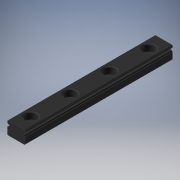
# Autodesk Inventor part: C-MLG9-75_r
Saved by Autodesk Inventor 2019 (Build 230136000, 136)
## iProperties
Created: 2023-11-06
Part Number: C-MLG9-75_r
Material: Generic
Catalog Web Link: www.cadenas.de
Description: C-MLG, E-GMLG_rail-Economy Miniature Liner guide - Standard type
Vendor: MISUMI
Document SubType Name: Modeling
Designer: psAdmin
Manufacturer: MISUMI
Mass: 3.65448 g
Surface Area: 29.3453 cm^2
Volume: 3.65448 cm^3
Density: 1 g/cm^3
Appearance: PSOLRGB-175-175-175
Category: PARTsolutions
Company: MISUMI
Title: C-MLG9-75
Author: Cadenas PARTsolutions
Comments: Economy Miniature Liner guide - Standard type
PSOL_IDENT_0: {$CADENAS_DATA/23d-libs/misumi/metric/06_linear_guides/c_mlg/c_mlg_rail.prj},214 {VTYP=3D},{NB=C-MLG
PSOL_IDENT_1: 9-75_r},{LINA=C-MLG9-75},{NN=C-MLG, E-GMLG_rail},{DATE=31.10.2023 10:57:24},{GEOMDATE=24.08.2023 00:
PSOL_IDENT_2: 31:00},{VERSION=},{LINEID=20},{WBVAR=ST,L,ALT1,ALT2,ALT3,ALT4,ES,ALT5,EB},{WBNUMERIC=L,ES,EB}  {NB=C
PSOL_IDENT_3: -MLG9-75_r},{LINA=C-MLG9-75},{KT=DUMMY},{PN=C-MLG9-75},{TYPE=C-MLG},{ST=1},{NM=9},{L=75},{LALG=[35:9
PSOL_IDENT_4: 00/1]},{H=10},{H1=2.0},{N=5.5},{W=20},{B=15},{B1=2.5},{C=10},{L1=17.5},{L2=29.60},{GNN=Dia.1.4},{MXL=
PSOL_IDENT_5: M3*3},{H2=1.8},{WRR=9},{HRR=6.5},{D=6.0},{HH=3.5},{DD=3.6},{P=20},{M=4},{E=7.5},{ALT1=},{ALT13D=4},{
PSOL_IDENT_6: ALT2=},{ALT3=},{ALT4=},{ES=0.0},{ESALG=0},{ESMIN=2.000},{ESMAX=13.000},{LE=7.5},{ALT4PN=},{ALT5=},{A
PSOL_IDENT_7: LT5ALG='','w/o EB (Right end face E size specification)','EB','with EB (Right end face E size specif
PSOL_IDENT_8: ication)' },{EB=0.0},{EBALG=0},{EBMIN=2.000},{EBMAX=13.000},{RE=7.5},{ALT5PN=},{NA=3},{R=1.00},{R1=0
PSOL_IDENT_9: .400},{C1=0.30},{WR1=0.4},{WR2=0.92},{WR3=0.38},{HR1=4.5},{L3D=75.0},{CID=6.000},{CIM=4.000}
NB: C-MLG9-75_r
NN: C-MLG, E-GMLG_rail
NT: Economy Miniature Liner guide - Standard type
NBSYN: $PN._r
LINA: C-MLG9-75
CATALOG: Misumi
PN: C-MLG9-75
ST: No Surface Treatment
L: 75
H: 10
H1: 2
N: 5.5
W: 20
B: 15
B1: 2.5
C: 10
L1: 17.5
L2: 29.6
GNN: Dia.1.4
MXL: M3*3
H2: 1.8
WRR: 9
HRR: 6.5
D: 6
HH: 3.5
DD: 3.6
P: 20
E: 7.5
ALT1: w/o MC (Tapped Holes)
ALT2: w/o (Additional Blocks)
ALT3: w/o Z1 (Pressure Change)
ALT4: w/o ES (Left end face E size specification)
ES: 0
ALT5: w/o EB (Right end face E size specification)
EB: 0
SUPPLIER: MISUMI
ARTICLENO: C-MLG9-75_r
BOMINFO: C-MLG9-75
CREATOR: CADENAS GmbH
Autodesk Inventor part; units mm, degrees
sketch "_____1" plane through (0, 0, 0) normal (0, 0, 1) x (1, 0, 0)
  line L0 (-4.5, 2.95) -> (-4.5, 2.1665)
  arc A0 (-3.9835, 1.65) -> (-4.5, 2.1665) centre (-4.9, 1.25) ccw
  line L1 (-3.9835, 1.65) -> (-3.6, 1.65)
  arc A1 (-3.6, 0.85) -> (-3.6, 1.65) centre (-3.6, 1.25) ccw
  line L2 (-3.6, 0.85) -> (-3.9835, 0.85)
  arc A2 (-4.5, 0.3335) -> (-3.9835, 0.85) centre (-4.9, 1.25) ccw
  line L3 (-4.5, 0.3335) -> (-4.5, -2.95)
  line L4 (-4.5, -2.95) -> (-4.2, -3.25)
  line L5 (-4.2, -3.25) -> (4.2, -3.25)
  line L6 (4.2, -3.25) -> (4.5, -2.95)
  line L7 (4.5, -2.95) -> (4.5, 0.3335)
  arc A3 (3.9835, 0.85) -> (4.5, 0.3335) centre (4.9, 1.25) ccw
  line L8 (3.9835, 0.85) -> (3.6, 0.85)
  arc A4 (3.6, 1.65) -> (3.6, 0.85) centre (3.6, 1.25) ccw
  line L9 (3.6, 1.65) -> (3.9835, 1.65)
  arc A5 (4.5, 2.1665) -> (3.9835, 1.65) centre (4.9, 1.25) ccw
  line L10 (4.5, 2.1665) -> (4.5, 2.95)
  line L11 (4.5, 2.95) -> (4.2, 3.25)
  line L12 (4.2, 3.25) -> (-4.2, 3.25)
  line L13 (-4.2, 3.25) -> (-4.5, 2.95)
  constraints: 28 end point, 12 point on circle, 6 centre point
extrude "Extrusion1" add sketch "_____1" along normal mid plane 75
sketch "_____5" plane through (0, 0, 30) normal (0, 0, 1) x (1, 0, 0)
  line L0 (0, 3.25) -> (0, -3.25)
  line L1 (0, -3.25) -> (-2.1, -3.25)
  line L2 (-2.1, -3.25) -> (-1.8, -2.95)
  line L3 (-1.8, -2.95) -> (-1.8, -0.25)
  line L4 (-1.8, -0.25) -> (-3, -0.25)
  line L5 (-3, -0.25) -> (-3, 2.95)
  line L6 (-3, 2.95) -> (-3.3, 3.25)
  line L7 (-3.3, 3.25) -> (0, 3.25)
  line L8 (0, 3.25) -> (0, -3.25)
  constraints: 18 end point
revolve "Revolution1" cut sketch "_____5" angle 360 about axis through (0, 3.25, 30) along (0, 1, 0)
pattern_linear "Rectangular Pattern1" count 4 spacing 20 along (0, 0, -1) of "Revolution1"
ref_plane "to_block1_XY" through (0, -3.25, 0) normal (0, 0, 1) x (1, 0, 0)
ref_plane "to_block1_YZ" through (0, -3.25, 0) normal (1, 0, 0) x (0, 1, 0)
ref_plane "to_block1_ZX" through (0, -3.25, 0) normal (0, 1, 0) x (0, 0, 1)
body "Solid1"
